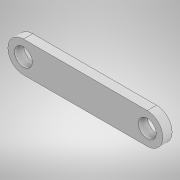
# Autodesk Inventor part: oled 고정대
Saved by Autodesk Inventor 2022 (Build 260153000, 153)
## iProperties
Created: 2024-07-09
Part Number: oled 고정대
Material: 일반
Document SubType Name: Modeling
Designer: seama
Density: 1 g/cm^3
Appearance: 기본값
Author: seama
Autodesk Inventor part; units mm, degrees
ref_plane "우측면도" through (0, 0, 0) normal (1, 0, 0) x (0, 1, 0)
ref_plane "평면도" through (0, 0, 0) normal (0, 1, 0) x (-1, 0, 0)
ref_plane "정면도" through (0, 0, 0) normal (0, 0, 1) x (1, 0, 0)
sketch "스케치1" plane through (0, 0, 0) normal (0, 0, 1) x (1, 0, 0)
  circle A0 centre (0, 0) radius 1.15
  circle A1 centre (16, 0) radius 1.15
  line L0 (0, 0) -> (16, 0) construction
  line L1 (0, -2) -> (16, -2)
  line L2 (16, 2) -> (0, 2)
  arc A2 (0, 2) -> (0, -2) centre (0, 0) ccw
  arc A3 (16, -2) -> (16, 2) centre (16, 0) ccw
  point P0 (8, 0)
  dimension "d0" = 16
  dimension "d1" = 2.3
  dimension "d3" = 2
  constraints: 8 end point, 4 centre point, 4 point on circle, 4 tangent, 1 coincident, 1 equal radius, 1 horizontal, 1 horizontal alignment, 1 midpoint, 1 parallel
  measures "d0" distance of L0.end point (0, 0)
  measures "d1" diameter of A0
  measures "d3" radius of A3
extrude "돌출1" add sketch "스케치1" against normal blind 1.2
